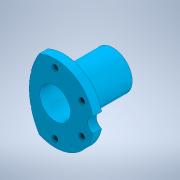
# Autodesk Inventor part: insertToScope
Saved by Autodesk Inventor 2022.1 (Build 261234020, 234B)
## iProperties
Created: 2020-09-09
Part Number: insertToScope
Material: PET Plastic
Document SubType Name: Modeling
Designer: robst
Density: 1.541 g/cm^3
Appearance: Sky Blue Medium
Author: robst
Autodesk Inventor part; units mm, degrees
ref_plane "YZ Plane" through (0, 0, 0) normal (1, 0, 0) x (0, 1, 0)
ref_plane "XZ Plane" through (0, 0, 0) normal (0, 1, 0) x (-1, 0, 0)
ref_plane "XY Plane" through (0, 0, 0) normal (0, 0, 1) x (1, 0, 0)
sketch "Sketch1" plane through (0, 0, 0) normal (0, 0, 1) x (1, 0, 0)
  circle A0 centre (0, 0) radius 15.875
  circle A1 centre (0, 0) radius 12.7
  dimension "d0" = 31.75
  dimension "d1" = 25.4
  constraints: 2 centre point, 2 coincident
  measures "d0" diameter of A0
  measures "d1" diameter of A1
extrude "Eyepiece Extrusion" add sketch "Sketch1" against normal blind 40.64
sketch "Sketch2" plane through (0, 0, 0) normal (0, 0, 1) x (1, 0, 0)
  circle A0 centre (0, 0) radius 12.7
  circle A1 centre (0, 0) radius 31.75
  dimension "d6" = 25.4
  dimension "d7" = 63.5
  constraints: 2 centre point, 2 coincident
  measures "d6" diameter of A0
  measures "d7" diameter of A1
extrude "Bolt Extrusion" add sketch "Sketch2" along normal blind 7.1374
sketch "Sketch3" plane through (0, 0, 0) normal (0, 0, -1) x (-1, 0, 0)
  circle A0 centre (0, 0) radius 31.75 projected
  circle A1 centre (-33.1656, 0) radius 54.6286 projected
  circle A2 centre (0, 0) radius 12.7 projected
  circle A3 centre (0, 0) radius 15.875 projected
  arc A4 (18.442, -17.4658) -> (18.442, 17.4658) centre (-33.1656, 0) ccw
  circle A5 centre (0, 0) radius 25.4 construction
  point P0 (13.2104, 28.8712)
  point P1 (13.2104, -28.8712)
  dimension "d8" = 108.966
  constraints: 4 point on circle, 2 centre point, 2 coincident
  measures "d8" diameter of A4
extrude "Cutout For Filter Wheel" cut sketch "Sketch3" against normal through all contours A0 A1 picked at (24.3045, -5.7561)
sketch "Sketch8" plane through (0, 0, 7.1374) normal (0, 0, 1) x (1, 0, 0)
  circle A0 centre (33.1724, 0) radius 6.35
  point P0 (0, 0)
  dimension "d50" = 12.7
  dimension "d51" = 33.1724
  constraints: 1 centre point
  measures "d50" diameter of A0
  measures "d51" distance of A0.centre point (0, 0)
extrude "Extrusion4" cut sketch "Sketch8" against normal through all
sketch "Sketch9" plane through (0, 0, 0) normal (0, 0, -1) x (-1, 0, 0)
  point P0 (0, 0)
  point P1 (0, 25.4)
  dimension "d59" = 25.4
  measures "d59" distance of point (0, 25.4) point (0, 0)
hole "Hole4" at (0, 25.4, 0) direction (0, 0, 1) diameter 4.699 depth 7.1374 counterbore diameter 5.5372 counterbore depth 5.5524
pattern_circular "Circular Pattern2" count 6 over 360 about axis through (0, 0, -10) along (0, 0, 1) of "Hole4"
equation "\"d0\" = outsideDiameter"
equation "\"d1\" = insideDiameter"
equation "\"d2\" = extrusionNoseDepth"
equation "\"d6\" = insideDiameter"
equation "\"d7\" = maxOutsideDiameter"
equation "\"d4\" = support"
equation "\"d59\" = radiusForHoles"
equation "\"outsideDiameter\" = 31.75"
equation "\"insideDiameter\" = 25.4"
equation "\"support\" = 7.1374"
equation "\"totalHeight\" = 44.45"
equation "\"maxOutsideDiameter\" = 63.5"
equation "\"eyepieceNoseDepth\" = 38.1"
equation "\"baseDepth\" = 2.54"
equation "\"extrusionNoseDepth\" = eyepieceNoseDepth + baseDepth"
equation "\"radiusForHoles\" = 25.4"
body "Solid1"
